Autodesk Fusion 360 part; units mm, degrees
(part 4 of 5)
  spline S17 degree 5 poles (-28.0678, -2.6304) (-28.0819, -2.6317) (-28.1102, -2.634) (-28.1526, -2.6363) (-28.2093, -2.6371) (-28.2803, -2.6353) (-28.3513, -2.6314) (-28.4224, -2.6261) (-28.4935, -2.6201) (-28.5647, -2.6137) (-28.6359, -2.6067) (-28.7071, -2.5991) (-28.7783, -2.5906) (-28.8495, -2.5811) (-28.9207, -2.5705) (-28.9919, -2.559) (-29.0631, -2.5467) (-29.1343, -2.5337) (-29.2055, -2.5201) (-29.2767, -2.5059) (-29.3478, -2.4912) (-29.419, -2.4759) (-29.4901, -2.46) (-29.5612, -2.4434) (-29.6322, -2.4261) (-29.7033, -2.4083) (-29.7743, -2.3899) (-29.8453, -2.3709) (-29.9162, -2.3515) (-29.9871, -2.3314) (-30.058, -2.3109) (-30.1288, -2.2899) (-30.1996, -2.2683) (-30.2704, -2.2463) (-30.3411, -2.2237) (-30.4117, -2.2006) (-30.4824, -2.1771) (-30.5529, -2.153) (-30.6235, -2.1285) (-30.6939, -2.1035) (-30.7644, -2.0781) (-30.8347, -2.0522) (-30.905, -2.0259) (-30.9753, -1.9991) (-31.0455, -1.9718) (-31.1156, -1.9441) (-31.1857, -1.916) (-31.2558, -1.8874) (-31.3257, -1.8584) (-31.3956, -1.829) (-31.4655, -1.7992) (-31.5352, -1.7689) (-31.6049, -1.7383) (-31.6746, -1.7072) (-31.7442, -1.6757) (-31.8137, -1.6438) (-31.8831, -1.6115) (-31.9524, -1.5788) (-32.0217, -1.5457) (-32.0909, -1.5122) (-32.1601, -1.4784) (-32.2291, -1.4441) (-32.2981, -1.4094) (-32.367, -1.3744) (-32.4359, -1.339) (-32.5046, -1.3032) (-32.5733, -1.267) (-32.6419, -1.2305) (-32.7104, -1.1936) (-32.7788, -1.1563) (-32.8471, -1.1186) (-32.9017, -1.0882) (-32.9427, -1.0652) (-32.9699, -1.0499) (-32.9835, -1.0421) knots 0 0 0 0 0 0 0.01428571 0.02857143 0.04285714 0.05714286 0.07142857 0.08571429 0.1 0.11428571 0.12857143 0.14285714 0.15714286 0.17142857 0.18571429 0.2 0.21428571 0.22857143 0.24285714 0.25714286 0.27142857 0.28571429 0.3 0.31428571 0.32857143 0.34285714 0.35714286 0.37142857 0.38571429 0.4 0.41428571 0.42857143 0.44285714 0.45714286 0.47142857 0.48571429 0.5 0.51428571 0.52857143 0.54285714 0.55714286 0.57142857 0.58571429 0.6 0.61428571 0.62857143 0.64285714 0.65714286 0.67142857 0.68571429 0.7 0.71428571 0.72857143 0.74285714 0.75714286 0.77142857 0.78571429 0.8 0.81428571 0.82857143 0.84285714 0.85714286 0.87142857 0.88571429 0.9 0.91428571 0.92857143 0.94285714 0.95714286 0.97142857 0.98571429 1 1 1 1 1 1
  line L17 (-28.0678, -2.6304) -> (-27.7691, -2.6026)
  arc A34 (-26.0521, -3.9455) -> (-27.7691, -2.6026) centre (-27.6217, -4.1832) ccw
  arc A35 (-26.0521, -3.9455) -> (-25.9963, -4.2981) centre (0, 0) ccw
  arc A36 (-27.2142, -6.1059) -> (-25.9963, -4.2981) centre (-27.5625, -4.5571) ccw
  line L18 (-27.2142, -6.1059) -> (-27.5069, -6.1717)
  spline S18 degree 5 poles (-27.5069, -6.1717) (-27.5207, -6.1748) (-27.5483, -6.1814) (-27.5894, -6.1924) (-27.6436, -6.2091) (-27.7105, -6.2328) (-27.7768, -6.2585) (-27.8428, -6.2854) (-27.9086, -6.3131) (-27.9743, -6.3412) (-28.0399, -6.3698) (-28.1052, -6.3991) (-28.1703, -6.4291) (-28.2351, -6.4602) (-28.2996, -6.4923) (-28.3637, -6.5252) (-28.4276, -6.5589) (-28.4913, -6.5933) (-28.5548, -6.6282) (-28.6182, -6.6637) (-28.6813, -6.6997) (-28.7442, -6.7362) (-28.8069, -6.7734) (-28.8694, -6.8111) (-28.9317, -6.8495) (-28.9937, -6.8884) (-29.0556, -6.9278) (-29.1172, -6.9678) (-29.1786, -7.0083) (-29.2399, -7.0492) (-29.301, -7.0906) (-29.3618, -7.1325) (-29.4225, -7.1749) (-29.483, -7.2177) (-29.5432, -7.261) (-29.6033, -7.3048) (-29.6632, -7.3491) (-29.7229, -7.3937) (-29.7824, -7.4388) (-29.8417, -7.4844) (-29.9008, -7.5303) (-29.9597, -7.5767) (-30.0185, -7.6235) (-30.077, -7.6707) (-30.1353, -7.7183) (-30.1935, -7.7663) (-30.2515, -7.8147) (-30.3092, -7.8635) (-30.3668, -7.9127) (-30.4242, -7.9623) (-30.4814, -8.0122) (-30.5384, -8.0626) (-30.5952, -8.1133) (-30.6519, -8.1644) (-30.7083, -8.2158) (-30.7645, -8.2676) (-30.8206, -8.3198) (-30.8765, -8.3723) (-30.9321, -8.4252) (-30.9876, -8.4784) (-31.0429, -8.532) (-31.098, -8.5859) (-31.1529, -8.6402) (-31.2076, -8.6948) (-31.2621, -8.7498) (-31.3164, -8.8051) (-31.3706, -8.8607) (-31.4245, -8.9166) (-31.4783, -8.9729) (-31.5318, -9.0295) (-31.5852, -9.0864) (-31.6277, -9.1322) (-31.6595, -9.1667) (-31.6807, -9.1898) (-31.6913, -9.2013) knots 0 0 0 0 0 0 0.01428571 0.02857143 0.04285714 0.05714286 0.07142857 0.08571429 0.1 0.11428571 0.12857143 0.14285714 0.15714286 0.17142857 0.18571429 0.2 0.21428571 0.22857143 0.24285714 0.25714286 0.27142857 0.28571429 0.3 0.31428571 0.32857143 0.34285714 0.35714286 0.37142857 0.38571429 0.4 0.41428571 0.42857143 0.44285714 0.45714286 0.47142857 0.48571429 0.5 0.51428571 0.52857143 0.54285714 0.55714286 0.57142857 0.58571429 0.6 0.61428571 0.62857143 0.64285714 0.65714286 0.67142857 0.68571429 0.7 0.71428571 0.72857143 0.74285714 0.75714286 0.77142857 0.78571429 0.8 0.81428571 0.82857143 0.84285714 0.85714286 0.87142857 0.88571429 0.9 0.91428571 0.92857143 0.94285714 0.95714286 0.97142857 0.98571429 1 1 1 1 1 1
  arc A37 (-31.6913, -9.2013) -> (-31.0472, -11.1836) centre (0, 0) ccw
  spline S19 degree 5 poles (-25.8812, -11.1751) (-25.8942, -11.1807) (-25.9204, -11.1916) (-25.9601, -11.2069) (-26.0137, -11.2252) (-26.0818, -11.2454) (-26.1506, -11.2636) (-26.2198, -11.2806) (-26.2893, -11.2969) (-26.359, -11.3128) (-26.4288, -11.3281) (-26.4989, -11.3429) (-26.5692, -11.3568) (-26.6399, -11.3697) (-26.7109, -11.3817) (-26.7822, -11.3928) (-26.8537, -11.4031) (-26.9254, -11.4127) (-26.9973, -11.4218) (-27.0694, -11.4303) (-27.1416, -11.4383) (-27.214, -11.4457) (-27.2866, -11.4525) (-27.3593, -11.4587) (-27.4322, -11.4643) (-27.5053, -11.4693) (-27.5785, -11.4737) (-27.6519, -11.4776) (-27.7254, -11.481) (-27.799, -11.4839) (-27.8727, -11.4863) (-27.9466, -11.4881) (-28.0206, -11.4895) (-28.0947, -11.4904) (-28.1689, -11.4908) (-28.2433, -11.4907) (-28.3177, -11.4901) (-28.3922, -11.489) (-28.4669, -11.4875) (-28.5416, -11.4855) (-28.6165, -11.4831) (-28.6914, -11.4802) (-28.7664, -11.4769) (-28.8415, -11.4731) (-28.9167, -11.4689) (-28.992, -11.4642) (-29.0673, -11.4591) (-29.1427, -11.4536) (-29.2182, -11.4477) (-29.2938, -11.4413) (-29.3695, -11.4345) (-29.4452, -11.4273) (-29.5209, -11.4196) (-29.5968, -11.4116) (-29.6727, -11.4032) (-29.7486, -11.3943) (-29.8246, -11.385) (-29.9007, -11.3754) (-29.9768, -11.3653) (-30.053, -11.3549) (-30.1292, -11.344) (-30.2055, -11.3328) (-30.2818, -11.3211) (-30.3582, -11.3091) (-30.4346, -11.2967) (-30.511, -11.2839) (-30.5875, -11.2707) (-30.664, -11.2572) (-30.7406, -11.2432) (-30.8172, -11.2289) (-30.8938, -11.2142) (-30.9551, -11.2022) (-31.0011, -11.193) (-31.0318, -11.1867) (-31.0472, -11.1836) knots 0 0 0 0 0 0 0.01428571 0.02857143 0.04285714 0.05714286 0.07142857 0.08571429 0.1 0.11428571 0.12857143 0.14285714 0.15714286 0.17142857 0.18571429 0.2 0.21428571 0.22857143 0.24285714 0.25714286 0.27142857 0.28571429 0.3 0.31428571 0.32857143 0.34285714 0.35714286 0.37142857 0.38571429 0.4 0.41428571 0.42857143 0.44285714 0.45714286 0.47142857 0.48571429 0.5 0.51428571 0.52857143 0.54285714 0.55714286 0.57142857 0.58571429 0.6 0.61428571 0.62857143 0.64285714 0.65714286 0.67142857 0.68571429 0.7 0.71428571 0.72857143 0.74285714 0.75714286 0.77142857 0.78571429 0.8 0.81428571 0.82857143 0.84285714 0.85714286 0.87142857 0.88571429 0.9 0.91428571 0.92857143 0.94285714 0.95714286 0.97142857 0.98571429 1 1 1 1 1 1
  line L19 (-25.8812, -11.1751) -> (-25.6057, -11.0563)
  arc A38 (-23.5578, -11.803) -> (-25.6057, -11.0563) centre (-24.9771, -12.5141) ccw
  arc A39 (-23.5578, -11.803) -> (-23.3957, -12.1211) centre (0, 0) ccw
  arc A40 (-23.9954, -14.2167) -> (-23.3957, -12.1211) centre (-24.8053, -12.8513) ccw
  line L20 (-23.9954, -14.2167) -> (-24.2534, -14.3698)
  spline S20 degree 5 poles (-24.2534, -14.3698) (-24.2657, -14.377) (-24.2899, -14.3918) (-24.3255, -14.4149) (-24.3719, -14.4475) (-24.4282, -14.4907) (-24.4834, -14.5357) (-24.5378, -14.5817) (-24.5918, -14.6283) (-24.6456, -14.6754) (-24.6991, -14.7228) (-24.7522, -14.7709) (-24.8048, -14.8196) (-24.8568, -14.8691) (-24.9083, -14.9195) (-24.9591, -14.9707) (-25.0095, -15.0225) (-25.0594, -15.0749) (-25.109, -15.1278) (-25.1583, -15.1811) (-25.2072, -15.2348) (-25.2557, -15.289) (-25.3039, -15.3437) (-25.3517, -15.3989) (-25.399, -15.4546) (-25.446, -15.5108) (-25.4927, -15.5674) (-25.5389, -15.6245) (-25.5849, -15.6819) (-25.6305, -15.7398) (-25.6758, -15.7981) (-25.7207, -15.8567) (-25.7653, -15.9158) (-25.8096, -15.9752) (-25.8535, -16.035) (-25.8971, -16.0952) (-25.9404, -16.1558) (-25.9834, -16.2167) (-26.026, -16.278) (-26.0683, -16.3396) (-26.1104, -16.4016) (-26.1521, -16.4639) (-26.1935, -16.5266) (-26.2346, -16.5896) (-26.2753, -16.6529) (-26.3158, -16.7165) (-26.356, -16.7804) (-26.3958, -16.8447) (-26.4354, -16.9093) (-26.4747, -16.9742) (-26.5136, -17.0394) (-26.5523, -17.1048) (-26.5907, -17.1706) (-26.6287, -17.2367) (-26.6665, -17.3031) (-26.704, -17.3697) (-26.7412, -17.4367) (-26.7781, -17.5039) (-26.8147, -17.5714) (-26.851, -17.6392) (-26.887, -17.7072) (-26.9227, -17.7755) (-26.9582, -17.8441) (-26.9933, -17.913) (-27.0282, -17.9821) (-27.0628, -18.0514) (-27.0971, -18.1211) (-27.1311, -18.1909) (-27.1648, -18.2611) (-27.1983, -18.3314) (-27.2314, -18.4021) (-27.2577, -18.4588) (-27.2773, -18.5014) (-27.2903, -18.5299) (-27.2968, -18.5441) knots 0 0 0 0 0 0 0.01428571 0.02857143 0.04285714 0.05714286 0.07142857 0.08571429 0.1 0.11428571 0.12857143 0.14285714 0.15714286 0.17142857 0.18571429 0.2 0.21428571 0.22857143 0.24285714 0.25714286 0.27142857 0.28571429 0.3 0.31428571 0.32857143 0.34285714 0.35714286 0.37142857 0.38571429 0.4 0.41428571 0.42857143 0.44285714 0.45714286 0.47142857 0.48571429 0.5 0.51428571 0.52857143 0.54285714 0.55714286 0.57142857 0.58571429 0.6 0.61428571 0.62857143 0.64285714 0.65714286 0.67142857 0.68571429 0.7 0.71428571 0.72857143 0.74285714 0.75714286 0.77142857 0.78571429 0.8 0.81428571 0.82857143 0.84285714 0.85714286 0.87142857 0.88571429 0.9 0.91428571 0.92857143 0.94285714 0.95714286 0.97142857 0.98571429 1 1 1 1 1 1
  arc A41 (-27.2968, -18.5441) -> (-26.0717, -20.2304) centre (0, 0) ccw
  spline S21 degree 5 poles (-21.1612, -18.6259) (-21.1718, -18.6353) (-21.1934, -18.6537) (-21.2264, -18.6805) (-21.2717, -18.7145) (-21.3302, -18.7547) (-21.39, -18.7933) (-21.4506, -18.8308) (-21.5117, -18.8678) (-21.573, -18.9044) (-21.6347, -18.9407) (-21.6968, -18.9763) (-21.7594, -19.0113) (-21.8226, -19.0454) (-21.8864, -19.0788) (-21.9508, -19.1113) (-22.0156, -19.1432) (-22.0809, -19.1745) (-22.1465, -19.2054) (-22.2124, -19.2358) (-22.2786, -19.2657) (-22.3452, -19.2951) (-22.4121, -19.324) (-22.4793, -19.3523) (-22.5469, -19.3802) (-22.6149, -19.4075) (-22.6832, -19.4344) (-22.7517, -19.4607) (-22.8206, -19.4867) (-22.8897, -19.5122) (-22.9591, -19.5372) (-23.0288, -19.5618) (-23.0987, -19.586) (-23.1689, -19.6098) (-23.2394, -19.6331) (-23.3101, -19.6559) (-23.3811, -19.6784) (-23.4523, -19.7004) (-23.5238, -19.722) (-23.5955, -19.7432) (-23.6674, -19.7641) (-23.7396, -19.7845) (-23.8119, -19.8045) (-23.8845, -19.8241) (-23.9573, -19.8433) (-24.0304, -19.8621) (-24.1036, -19.8806) (-24.177, -19.8986) (-24.2507, -19.9163) (-24.3245, -19.9336) (-24.3986, -19.9505) (-24.4728, -19.967) (-24.5472, -19.9832) (-24.6218, -19.999) (-24.6966, -20.0144) (-24.7716, -20.0295) (-24.8467, -20.0441) (-24.9221, -20.0585) (-24.9976, -20.0724) (-25.0733, -20.086) (-25.1491, -20.0992) (-25.2251, -20.1121) (-25.3013, -20.1246) (-25.3776, -20.1368) (-25.4541, -20.1486) (-25.5308, -20.16) (-25.6076, -20.1711) (-25.6846, -20.1819) (-25.7617, -20.1923) (-25.839, -20.2024) (-25.9164, -20.2121) (-25.9784, -20.2196) (-26.025, -20.225) (-26.0561, -20.2286) (-26.0717, -20.2304) knots 0 0 0 0 0 0 0.01428571 0.02857143 0.04285714 0.05714286 0.07142857 0.08571429 0.1 0.11428571 0.12857143 0.14285714 0.15714286 0.17142857 0.18571429 0.2 0.21428571 0.22857143 0.24285714 0.25714286 0.27142857 0.28571429 0.3 0.31428571 0.32857143 0.34285714 0.35714286 0.37142857 0.38571429 0.4 0.41428571 0.42857143 0.44285714 0.45714286 0.47142857 0.48571429 0.5 0.51428571 0.52857143 0.54285714 0.55714286 0.57142857 0.58571429 0.6 0.61428571 0.62857143 0.64285714 0.65714286 0.67142857 0.68571429 0.7 0.71428571 0.72857143 0.74285714 0.75714286 0.77142857 0.78571429 0.8 0.81428571 0.82857143 0.84285714 0.85714286 0.87142857 0.88571429 0.9 0.91428571 0.92857143 0.94285714 0.95714286 0.97142857 0.98571429 1 1 1 1 1 1
  line L21 (-21.1612, -18.6259) -> (-20.9359, -18.4278)
  arc A42 (-18.7575, -18.5051) -> (-20.9359, -18.4278) centre (-19.8876, -19.62) ccw
  arc A43 (-18.7575, -18.5051) -> (-18.5051, -18.7575) centre (0, 0) ccw
  arc A44 (-18.4278, -20.9359) -> (-18.5051, -18.7575) centre (-19.62, -19.8876) ccw
  line L22 (-18.4278, -20.9359) -> (-18.6259, -21.1612)
  spline S22 degree 5 poles (-18.6259, -21.1612) (-18.6353, -21.1718) (-18.6537, -21.1934) (-18.6805, -21.2264) (-18.7145, -21.2717) (-18.7547, -21.3302) (-18.7933, -21.39) (-18.8308, -21.4506) (-18.8678, -21.5117) (-18.9044, -21.573) (-18.9407, -21.6347) (-18.9763, -21.6968) (-19.0113, -21.7594) (-19.0454, -21.8226) (-19.0788, -21.8864) (-19.1113, -21.9508) (-19.1432, -22.0156) (-19.1745, -22.0809) (-19.2054, -22.1465) (-19.2358, -22.2124) (-19.2657, -22.2786) (-19.2951, -22.3452) (-19.324, -22.4121) (-19.3523, -22.4793) (-19.3802, -22.5469) (-19.4075, -22.6149) (-19.4344, -22.6832) (-19.4607, -22.7517) (-19.4867, -22.8206) (-19.5122, -22.8897) (-19.5372, -22.9591) (-19.5618, -23.0288) (-19.586, -23.0987) (-19.6098, -23.1689) (-19.6331, -23.2394) (-19.6559, -23.3101) (-19.6784, -23.3811) (-19.7004, -23.4523) (-19.722, -23.5238) (-19.7432, -23.5955) (-19.7641, -23.6674) (-19.7845, -23.7396) (-19.8045, -23.8119) (-19.8241, -23.8845) (-19.8433, -23.9573) (-19.8621, -24.0304) (-19.8806, -24.1036) (-19.8986, -24.177) (-19.9163, -24.2507) (-19.9336, -24.3245) (-19.9505, -24.3986) (-19.967, -24.4728) (-19.9832, -24.5472) (-19.999, -24.6218) (-20.0144, -24.6966) (-20.0295, -24.7716) (-20.0441, -24.8467) (-20.0585, -24.9221) (-20.0724, -24.9976) (-20.086, -25.0733) (-20.0992, -25.1491) (-20.1121, -25.2251) (-20.1246, -25.3013) (-20.1368, -25.3776) (-20.1486, -25.4541) (-20.16, -25.5308) (-20.1711, -25.6076) (-20.1819, -25.6846) (-20.1923, -25.7617) (-20.2024, -25.839) (-20.2121, -25.9164) (-20.2196, -25.9784) (-20.225, -26.025) (-20.2286, -26.0561) (-20.2304, -26.0717) knots 0 0 0 0 0 0 0.01428571 0.02857143 0.04285714 0.05714286 0.07142857 0.08571429 0.1 0.11428571 0.12857143 0.14285714 0.15714286 0.17142857 0.18571429 0.2 0.21428571 0.22857143 0.24285714 0.25714286 0.27142857 0.28571429 0.3 0.31428571 0.32857143 0.34285714 0.35714286 0.37142857 0.38571429 0.4 0.41428571 0.42857143 0.44285714 0.45714286 0.47142857 0.48571429 0.5 0.51428571 0.52857143 0.54285714 0.55714286 0.57142857 0.58571429 0.6 0.61428571 0.62857143 0.64285714 0.65714286 0.67142857 0.68571429 0.7 0.71428571 0.72857143 0.74285714 0.75714286 0.77142857 0.78571429 0.8 0.81428571 0.82857143 0.84285714 0.85714286 0.87142857 0.88571429 0.9 0.91428571 0.92857143 0.94285714 0.95714286 0.97142857 0.98571429 1 1 1 1 1 1
  arc A45 (-20.2304, -26.0717) -> (-18.5441, -27.2968) centre (0, 0) ccw
  spline S23 degree 5 poles (-14.3698, -24.2534) (-14.377, -24.2657) (-14.3918, -24.2899) (-14.4149, -24.3255) (-14.4475, -24.3719) (-14.4907, -24.4282) (-14.5357, -24.4834) (-14.5817, -24.5378) (-14.6283, -24.5918) (-14.6754, -24.6456) (-14.7228, -24.6991) (-14.7709, -24.7522) (-14.8196, -24.8048) (-14.8691, -24.8568) (-14.9195, -24.9083) (-14.9707, -24.9591) (-15.0225, -25.0095) (-15.0749, -25.0594) (-15.1278, -25.109) (-15.1811, -25.1583) (-15.2348, -25.2072) (-15.289, -25.2557) (-15.3437, -25.3039) (-15.3989, -25.3517) (-15.4546, -25.399) (-15.5108, -25.446) (-15.5674, -25.4927) (-15.6245, -25.5389) (-15.6819, -25.5849) (-15.7398, -25.6305) (-15.7981, -25.6758) (-15.8567, -25.7207) (-15.9158, -25.7653) (-15.9752, -25.8096) (-16.035, -25.8535) (-16.0952, -25.8971) (-16.1558, -25.9404) (-16.2167, -25.9834) (-16.278, -26.026) (-16.3396, -26.0683) (-16.4016, -26.1104) (-16.4639, -26.1521) (-16.5266, -26.1935) (-16.5896, -26.2346) (-16.6529, -26.2753) (-16.7165, -26.3158) (-16.7804, -26.356) (-16.8447, -26.3958) (-16.9093, -26.4354) (-16.9742, -26.4747) (-17.0394, -26.5136) (-17.1048, -26.5523) (-17.1706, -26.5907) (-17.2367, -26.6287) (-17.3031, -26.6665) (-17.3697, -26.704) (-17.4367, -26.7412) (-17.5039, -26.7781) (-17.5714, -26.8147) (-17.6392, -26.851) (-17.7072, -26.887) (-17.7755, -26.9227) (-17.8441, -26.9582) (-17.913, -26.9933) (-17.9821, -27.0282) (-18.0514, -27.0628) (-18.1211, -27.0971) (-18.1909, -27.1311) (-18.2611, -27.1648) (-18.3314, -27.1983) (-18.4021, -27.2314) (-18.4588, -27.2577) (-18.5014, -27.2773) (-18.5299, -27.2903) (-18.5441, -27.2968) knots 0 0 0 0 0 0 0.01428571 0.02857143 0.04285714 0.05714286 0.07142857 0.08571429 0.1 0.11428571 0.12857143 0.14285714 0.15714286 0.17142857 0.18571429 0.2 0.21428571 0.22857143 0.24285714 0.25714286 0.27142857 0.28571429 0.3 0.31428571 0.32857143 0.34285714 0.35714286 0.37142857 0.38571429 0.4 0.41428571 0.42857143 0.44285714 0.45714286 0.47142857 0.48571429 0.5 0.51428571 0.52857143 0.54285714 0.55714286 0.57142857 0.58571429 0.6 0.61428571 0.62857143 0.64285714 0.65714286 0.67142857 0.68571429 0.7 0.71428571 0.72857143 0.74285714 0.75714286 0.77142857 0.78571429 0.8 0.81428571 0.82857143 0.84285714 0.85714286 0.87142857 0.88571429 0.9 0.91428571 0.92857143 0.94285714 0.95714286 0.97142857 0.98571429 1 1 1 1 1 1
  line L23 (-14.3698, -24.2534) -> (-14.2167, -23.9954)
  arc A46 (-12.1211, -23.3957) -> (-14.2167, -23.9954) centre (-12.8513, -24.8053) ccw
  arc A47 (-12.1211, -23.3957) -> (-11.803, -23.5578) centre (0, 0) ccw
  arc A48 (-11.0563, -25.6057) -> (-11.803, -23.5578) centre (-12.5141, -24.9771) ccw
  line L24 (-11.0563, -25.6057) -> (-11.1751, -25.8812)
  spline S24 degree 5 poles (-11.1751, -25.8812) (-11.1807, -25.8942) (-11.1916, -25.9204) (-11.2069, -25.9601) (-11.2252, -26.0137) (-11.2454, -26.0818) (-11.2636, -26.1506) (-11.2806, -26.2198) (-11.2969, -26.2893) (-11.3128, -26.359) (-11.3281, -26.4288) (-11.3429, -26.4989) (-11.3568, -26.5692) (-11.3697, -26.6399) (-11.3817, -26.7109) (-11.3928, -26.7822) (-11.4031, -26.8537) (-11.4127, -26.9254) (-11.4218, -26.9973) (-11.4303, -27.0694) (-11.4383, -27.1416) (-11.4457, -27.214) (-11.4525, -27.2866) (-11.4587, -27.3593) (-11.4643, -27.4322) (-11.4693, -27.5053) (-11.4737, -27.5785) (-11.4776, -27.6519) (-11.481, -27.7254) (-11.4839, -27.799) (-11.4863, -27.8727) (-11.4881, -27.9466) (-11.4895, -28.0206) (-11.4904, -28.0947) (-11.4908, -28.1689) (-11.4907, -28.2433) (-11.4901, -28.3177) (-11.489, -28.3922) (-11.4875, -28.4669) (-11.4855, -28.5416) (-11.4831, -28.6165) (-11.4802, -28.6914) (-11.4769, -28.7664) (-11.4731, -28.8415) (-11.4689, -28.9167) (-11.4642, -28.992) (-11.4591, -29.0673) (-11.4536, -29.1427) (-11.4477, -29.2182) (-11.4413, -29.2938) (-11.4345, -29.3695) (-11.4273, -29.4452) (-11.4196, -29.5209) (-11.4116, -29.5968) (-11.4032, -29.6727) (-11.3943, -29.7486) (-11.385, -29.8246) (-11.3754, -29.9007) (-11.3653, -29.9768) (-11.3549, -30.053) (-11.344, -30.1292) (-11.3328, -30.2055) (-11.3211, -30.2818) (-11.3091, -30.3582) (-11.2967, -30.4346) (-11.2839, -30.511) (-11.2707, -30.5875) (-11.2572, -30.664) (-11.2432, -30.7406) (-11.2289, -30.8172) (-11.2142, -30.8938) (-11.2022, -30.9551) (-11.193, -31.0011) (-11.1867, -31.0318) (-11.1836, -31.0472) knots 0 0 0 0 0 0 0.01428571 0.02857143 0.04285714 0.05714286 0.07142857 0.08571429 0.1 0.11428571 0.12857143 0.14285714 0.15714286 0.17142857 0.18571429 0.2 0.21428571 0.22857143 0.24285714 0.25714286 0.27142857 0.28571429 0.3 0.31428571 0.32857143 0.34285714 0.35714286 0.37142857 0.38571429 0.4 0.41428571 0.42857143 0.44285714 0.45714286 0.47142857 0.48571429 0.5 0.51428571 0.52857143 0.54285714 0.55714286 0.57142857 0.58571429 0.6 0.61428571 0.62857143 0.64285714 0.65714286 0.67142857 0.68571429 0.7 0.71428571 0.72857143 0.74285714 0.75714286 0.77142857 0.78571429 0.8 0.81428571 0.82857143 0.84285714 0.85714286 0.87142857 0.88571429 0.9 0.91428571 0.92857143 0.94285714 0.95714286 0.97142857 0.98571429 1 1 1 1 1 1
  arc A49 (-11.1836, -31.0472) -> (-9.2013, -31.6913) centre (0, 0) ccw
  spline S25 degree 5 poles (-6.1717, -27.5069) (-6.1748, -27.5207) (-6.1814, -27.5483) (-6.1924, -27.5894) (-6.2091, -27.6436) (-6.2328, -27.7105) (-6.2585, -27.7768) (-6.2854, -27.8428) (-6.3131, -27.9086) (-6.3412, -27.9743) (-6.3698, -28.0399) (-6.3991, -28.1052) (-6.4291, -28.1703) (-6.4602, -28.2351) (-6.4923, -28.2996) (-6.5252, -28.3637) (-6.5589, -28.4276) (-6.5933, -28.4913) (-6.6282, -28.5548) (-6.6637, -28.6182) (-6.6997, -28.6813) (-6.7362, -28.7442) (-6.7734, -28.8069) (-6.8111, -28.8694) (-6.8495, -28.9317) (-6.8884, -28.9937) (-6.9278, -29.0556) (-6.9678, -29.1172) (-7.0083, -29.1786) (-7.0492, -29.2399) (-7.0906, -29.301) (-7.1325, -29.3618) (-7.1749, -29.4225) (-7.2177, -29.483) (-7.261, -29.5432) (-7.3048, -29.6033) (-7.3491, -29.6632) (-7.3937, -29.7229) (-7.4388, -29.7824) (-7.4844, -29.8417) (-7.5303, -29.9008) (-7.5767, -29.9597) (-7.6235, -30.0185) (-7.6707, -30.077) (-7.7183, -30.1353) (-7.7663, -30.1935) (-7.8147, -30.2515) (-7.8635, -30.3092) (-7.9127, -30.3668) (-7.9623, -30.4242) (-8.0122, -30.4814) (-8.0626, -30.5384) (-8.1133, -30.5952) (-8.1644, -30.6519) (-8.2158, -30.7083) (-8.2676, -30.7645) (-8.3198, -30.8206) (-8.3723, -30.8765) (-8.4252, -30.9321) (-8.4784, -30.9876) (-8.532, -31.0429) (-8.5859, -31.098) (-8.6402, -31.1529) (-8.6948, -31.2076) (-8.7498, -31.2621) (-8.8051, -31.3164) (-8.8607, -31.3706) (-8.9166, -31.4245) (-8.9729, -31.4783) (-9.0295, -31.5318) (-9.0864, -31.5852) (-9.1322, -31.6277) (-9.1667, -31.6595) (-9.1898, -31.6807) (-9.2013, -31.6913) knots 0 0 0 0 0 0 0.01428571 0.02857143 0.04285714 0.05714286 0.07142857 0.08571429 0.1 0.11428571 0.12857143 0.14285714 0.15714286 0.17142857 0.18571429 0.2 0.21428571 0.22857143 0.24285714 0.25714286 0.27142857 0.28571429 0.3 0.31428571 0.32857143 0.34285714 0.35714286 0.37142857 0.38571429 0.4 0.41428571 0.42857143 0.44285714 0.45714286 0.47142857 0.48571429 0.5 0.51428571 0.52857143 0.54285714 0.55714286 0.57142857 0.58571429 0.6 0.61428571 0.62857143 0.64285714 0.65714286 0.67142857 0.68571429 0.7 0.71428571 0.72857143 0.74285714 0.75714286 0.77142857 0.78571429 0.8 0.81428571 0.82857143 0.84285714 0.85714286 0.87142857 0.88571429 0.9 0.91428571 0.92857143 0.94285714 0.95714286 0.97142857 0.98571429 1 1 1 1 1 1
  line L25 (-6.1717, -27.5069) -> (-6.1059, -27.2142)
  arc A50 (-4.2981, -25.9963) -> (-6.1059, -27.2142) centre (-4.5571, -27.5625) ccw
  arc A51 (-4.2981, -25.9963) -> (-3.9455, -26.0521) centre (0, 0) ccw
  arc A52 (-2.6026, -27.7691) -> (-3.9455, -26.0521) centre (-4.1832, -27.6217) ccw
  line L26 (-2.6026, -27.7691) -> (-2.6304, -28.0678)
  spline S26 degree 5 poles (-2.6304, -28.0678) (-2.6317, -28.0819) (-2.634, -28.1102) (-2.6363, -28.1526) (-2.6371, -28.2093) (-2.6353, -28.2803) (-2.6314, -28.3513) (-2.6261, -28.4224) (-2.6201, -28.4935) (-2.6137, -28.5647) (-2.6067, -28.6359) (-2.5991, -28.7071) (-2.5906, -28.7783) (-2.5811, -28.8495) (-2.5705, -28.9207) (-2.559, -28.9919) (-2.5467, -29.0631) (-2.5337, -29.1343) (-2.5201, -29.2055) (-2.5059, -29.2767) (-2.4912, -29.3478) (-2.4759, -29.419) (-2.46, -29.4901) (-2.4434, -29.5612) (-2.4261, -29.6322) (-2.4083, -29.7033) (-2.3899, -29.7743) (-2.3709, -29.8453) (-2.3515, -29.9162) (-2.3314, -29.9871) (-2.3109, -30.058) (-2.2899, -30.1288) (-2.2683, -30.1996) (-2.2463, -30.2704) (-2.2237, -30.3411) (-2.2006, -30.4117) (-2.1771, -30.4824) (-2.153, -30.5529) (-2.1285, -30.6235) (-2.1035, -30.6939) (-2.0781, -30.7644) (-2.0522, -30.8347) (-2.0259, -30.905) (-1.9991, -30.9753) (-1.9718, -31.0455) (-1.9441, -31.1156) (-1.916, -31.1857) (-1.8874, -31.2558) (-1.8584, -31.3257) (-1.829, -31.3956) (-1.7992, -31.4655) (-1.7689, -31.5352) (-1.7383, -31.6049) (-1.7072, -31.6746) (-1.6757, -31.7442) (-1.6438, -31.8137) (-1.6115, -31.8831) (-1.5788, -31.9524) (-1.5457, -32.0217) (-1.5122, -32.0909) (-1.4784, -32.1601) (-1.4441, -32.2291) (-1.4094, -32.2981) (-1.3744, -32.367) (-1.339, -32.4359) (-1.3032, -32.5046) (-1.267, -32.5733) (-1.2305, -32.6419) (-1.1936, -32.7104) (-1.1563, -32.7788) (-1.1186, -32.8471) (-1.0882, -32.9017) (-1.0652, -32.9427) (-1.0499, -32.9699) (-1.0421, -32.9835) knots 0 0 0 0 0 0 0.01428571 0.02857143 0.04285714 0.05714286 0.07142857 0.08571429 0.1 0.11428571 0.12857143 0.14285714 0.15714286 0.17142857 0.18571429 0.2 0.21428571 0.22857143 0.24285714 0.25714286 0.27142857 0.28571429 0.3 0.31428571 0.32857143 0.34285714 0.35714286 0.37142857 0.38571429 0.4 0.41428571 0.42857143 0.44285714 0.45714286 0.47142857 0.48571429 0.5 0.51428571 0.52857143 0.54285714 0.55714286 0.57142857 0.58571429 0.6 0.61428571 0.62857143 0.64285714 0.65714286 0.67142857 0.68571429 0.7 0.71428571 0.72857143 0.74285714 0.75714286 0.77142857 0.78571429 0.8 0.81428571 0.82857143 0.84285714 0.85714286 0.87142857 0.88571429 0.9 0.91428571 0.92857143 0.94285714 0.95714286 0.97142857 0.98571429 1 1 1 1 1 1
  arc A53 (-1.0421, -32.9835) -> (1.0421, -32.9835) centre (0, 0) ccw
  spline S27 degree 5 poles (2.6304, -28.0678) (2.6317, -28.0819) (2.634, -28.1102) (2.6363, -28.1526) (2.6371, -28.2093) (2.6353, -28.2803) (2.6314, -28.3513) (2.6261, -28.4224) (2.6201, -28.4935) (2.6137, -28.5647) (2.6067, -28.6359) (2.5991, -28.7071) (2.5906, -28.7783) (2.5811, -28.8495) (2.5705, -28.9207) (2.559, -28.9919) (2.5467, -29.0631) (2.5337, -29.1343) (2.5201, -29.2055) (2.5059, -29.2767) (2.4912, -29.3478) (2.4759, -29.419) (2.46, -29.4901) (2.4434, -29.5612) (2.4261, -29.6322) (2.4083, -29.7033) (2.3899, -29.7743) (2.3709, -29.8453) (2.3515, -29.9162) (2.3314, -29.9871) (2.3109, -30.058) (2.2899, -30.1288) (2.2683, -30.1996) (2.2463, -30.2704) (2.2237, -30.3411) (2.2006, -30.4117) (2.1771, -30.4824) (2.153, -30.5529) (2.1285, -30.6235) (2.1035, -30.6939) (2.0781, -30.7644) (2.0522, -30.8347) (2.0259, -30.905) (1.9991, -30.9753) (1.9718, -31.0455) (1.9441, -31.1156) (1.916, -31.1857) (1.8874, -31.2558) (1.8584, -31.3257) (1.829, -31.3956) (1.7992, -31.4655) (1.7689, -31.5352) (1.7383, -31.6049) (1.7072, -31.6746) (1.6757, -31.7442) (1.6438, -31.8137) (1.6115, -31.8831) (1.5788, -31.9524) (1.5457, -32.0217) (1.5122, -32.0909) (1.4784, -32.1601) (1.4441, -32.2291) (1.4094, -32.2981) (1.3744, -32.367) (1.339, -32.4359) (1.3032, -32.5046) (1.267, -32.5733) (1.2305, -32.6419) (1.1936, -32.7104) (1.1563, -32.7788) (1.1186, -32.8471) (1.0882, -32.9017) (1.0652, -32.9427) (1.0499, -32.9699) (1.0421, -32.9835) knots 0 0 0 0 0 0 0.01428571 0.02857143 0.04285714 0.05714286 0.07142857 0.08571429 0.1 0.11428571 0.12857143 0.14285714 0.15714286 0.17142857 0.18571429 0.2 0.21428571 0.22857143 0.24285714 0.25714286 0.27142857 0.28571429 0.3 0.31428571 0.32857143 0.34285714 0.35714286 0.37142857 0.38571429 0.4 0.41428571 0.42857143 0.44285714 0.45714286 0.47142857 0.48571429 0.5 0.51428571 0.52857143 0.54285714 0.55714286 0.57142857 0.58571429 0.6 0.61428571 0.62857143 0.64285714 0.65714286 0.67142857 0.68571429 0.7 0.71428571 0.72857143 0.74285714 0.75714286 0.77142857 0.78571429 0.8 0.81428571 0.82857143 0.84285714 0.85714286 0.87142857 0.88571429 0.9 0.91428571 0.92857143 0.94285714 0.95714286 0.97142857 0.98571429 1 1 1 1 1 1
  line L27 (2.6304, -28.0678) -> (2.6026, -27.7691)
  arc A54 (3.9455, -26.0521) -> (2.6026, -27.7691) centre (4.1832, -27.6217) ccw
  arc A55 (3.9455, -26.0521) -> (4.2981, -25.9963) centre (0, 0) ccw
  arc A56 (6.1059, -27.2142) -> (4.2981, -25.9963) centre (4.5571, -27.5625) ccw
  line L28 (6.1059, -27.2142) -> (6.1717, -27.5069)
  spline S28 degree 5 poles (6.1717, -27.5069) (6.1748, -27.5207) (6.1814, -27.5483) (6.1924, -27.5894) (6.2091, -27.6436) (6.2328, -27.7105) (6.2585, -27.7768) (6.2854, -27.8428) (6.3131, -27.9086) (6.3412, -27.9743) (6.3698, -28.0399) (6.3991, -28.1052) (6.4291, -28.1703) (6.4602, -28.2351) (6.4923, -28.2996) (6.5252, -28.3637) (6.5589, -28.4276) (6.5933, -28.4913) (6.6282, -28.5548) (6.6637, -28.6182) (6.6997, -28.6813) (6.7362, -28.7442) (6.7734, -28.8069) (6.8111, -28.8694) (6.8495, -28.9317) (6.8884, -28.9937) (6.9278, -29.0556) (6.9678, -29.1172) (7.0083, -29.1786) (7.0492, -29.2399) (7.0906, -29.301) (7.1325, -29.3618) (7.1749, -29.4225) (7.2177, -29.483) (7.261, -29.5432) (7.3048, -29.6033) (7.3491, -29.6632) (7.3937, -29.7229) (7.4388, -29.7824) (7.4844, -29.8417) (7.5303, -29.9008) (7.5767, -29.9597) (7.6235, -30.0185) (7.6707, -30.077) (7.7183, -30.1353) (7.7663, -30.1935) (7.8147, -30.2515) (7.8635, -30.3092) (7.9127, -30.3668) (7.9623, -30.4242) (8.0122, -30.4814) (8.0626, -30.5384) (8.1133, -30.5952) (8.1644, -30.6519) (8.2158, -30.7083) (8.2676, -30.7645) (8.3198, -30.8206) (8.3723, -30.8765) (8.4252, -30.9321) (8.4784, -30.9876) (8.532, -31.0429) (8.5859, -31.098) (8.6402, -31.1529) (8.6948, -31.2076) (8.7498, -31.2621) (8.8051, -31.3164) (8.8607, -31.3706) (8.9166, -31.4245) (8.9729, -31.4783) (9.0295, -31.5318) (9.0864, -31.5852) (9.1322, -31.6277) (9.1667, -31.6595) (9.1898, -31.6807) (9.2013, -31.6913) knots 0 0 0 0 0 0 0.01428571 0.02857143 0.04285714 0.05714286 0.07142857 0.08571429 0.1 0.11428571 0.12857143 0.14285714 0.15714286 0.17142857 0.18571429 0.2 0.21428571 0.22857143 0.24285714 0.25714286 0.27142857 0.28571429 0.3 0.31428571 0.32857143 0.34285714 0.35714286 0.37142857 0.38571429 0.4 0.41428571 0.42857143 0.44285714 0.45714286 0.47142857 0.48571429 0.5 0.51428571 0.52857143 0.54285714 0.55714286 0.57142857 0.58571429 0.6 0.61428571 0.62857143 0.64285714 0.65714286 0.67142857 0.68571429 0.7 0.71428571 0.72857143 0.74285714 0.75714286 0.77142857 0.78571429 0.8 0.81428571 0.82857143 0.84285714 0.85714286 0.87142857 0.88571429 0.9 0.91428571 0.92857143 0.94285714 0.95714286 0.97142857 0.98571429 1 1 1 1 1 1
  arc A57 (9.2013, -31.6913) -> (11.1836, -31.0472) centre (0, 0) ccw
  spline S29 degree 5 poles (11.1751, -25.8812) (11.1807, -25.8942) (11.1916, -25.9204) (11.2069, -25.9601) (11.2252, -26.0137) (11.2454, -26.0818) (11.2636, -26.1506) (11.2806, -26.2198) (11.2969, -26.2893) (11.3128, -26.359) (11.3281, -26.4288) (11.3429, -26.4989) (11.3568, -26.5692) (11.3697, -26.6399) (11.3817, -26.7109) (11.3928, -26.7822) (11.4031, -26.8537) (11.4127, -26.9254) (11.4218, -26.9973) (11.4303, -27.0694) (11.4383, -27.1416) (11.4457, -27.214) (11.4525, -27.2866) (11.4587, -27.3593) (11.4643, -27.4322) (11.4693, -27.5053) (11.4737, -27.5785) (11.4776, -27.6519) (11.481, -27.7254) (11.4839, -27.799) (11.4863, -27.8727) (11.4881, -27.9466) (11.4895, -28.0206) (11.4904, -28.0947) (11.4908, -28.1689) (11.4907, -28.2433) (11.4901, -28.3177) (11.489, -28.3922) (11.4875, -28.4669) (11.4855, -28.5416) (11.4831, -28.6165) (11.4802, -28.6914) (11.4769, -28.7664) (11.4731, -28.8415) (11.4689, -28.9167) (11.4642, -28.992) (11.4591, -29.0673) (11.4536, -29.1427) (11.4477, -29.2182) (11.4413, -29.2938) (11.4345, -29.3695) (11.4273, -29.4452) (11.4196, -29.5209) (11.4116, -29.5968) (11.4032, -29.6727) (11.3943, -29.7486) (11.385, -29.8246) (11.3754, -29.9007) (11.3653, -29.9768) (11.3549, -30.053) (11.344, -30.1292) (11.3328, -30.2055) (11.3211, -30.2818) (11.3091, -30.3582) (11.2967, -30.4346) (11.2839, -30.511) (11.2707, -30.5875) (11.2572, -30.664) (11.2432, -30.7406) (11.2289, -30.8172) (11.2142, -30.8938) (11.2022, -30.9551) (11.193, -31.0011) (11.1867, -31.0318) (11.1836, -31.0472) knots 0 0 0 0 0 0 0.01428571 0.02857143 0.04285714 0.05714286 0.07142857 0.08571429 0.1 0.11428571 0.12857143 0.14285714 0.15714286 0.17142857 0.18571429 0.2 0.21428571 0.22857143 0.24285714 0.25714286 0.27142857 0.28571429 0.3 0.31428571 0.32857143 0.34285714 0.35714286 0.37142857 0.38571429 0.4 0.41428571 0.42857143 0.44285714 0.45714286 0.47142857 0.48571429 0.5 0.51428571 0.52857143 0.54285714 0.55714286 0.57142857 0.58571429 0.6 0.61428571 0.62857143 0.64285714 0.65714286 0.67142857 0.68571429 0.7 0.71428571 0.72857143 0.74285714 0.75714286 0.77142857 0.78571429 0.8 0.81428571 0.82857143 0.84285714 0.85714286 0.87142857 0.88571429 0.9 0.91428571 0.92857143 0.94285714 0.95714286 0.97142857 0.98571429 1 1 1 1 1 1
  line L29 (11.1751, -25.8812) -> (11.0563, -25.6057)
  arc A58 (11.803, -23.5578) -> (11.0563, -25.6057) centre (12.5141, -24.9771) ccw
  arc A59 (11.803, -23.5578) -> (12.1211, -23.3957) centre (0, 0) ccw
  arc A60 (14.2167, -23.9954) -> (12.1211, -23.3957) centre (12.8513, -24.8053) ccw
  line L30 (14.2167, -23.9954) -> (14.3698, -24.2534)
  spline S30 degree 5 poles (14.3698, -24.2534) (14.377, -24.2657) (14.3918, -24.2899) (14.4149, -24.3255) (14.4475, -24.3719) (14.4907, -24.4282) (14.5357, -24.4834) (14.5817, -24.5378) (14.6283, -24.5918) (14.6754, -24.6456) (14.7228, -24.6991) (14.7709, -24.7522) (14.8196, -24.8048) (14.8691, -24.8568) (14.9195, -24.9083) (14.9707, -24.9591) (15.0225, -25.0095) (15.0749, -25.0594) (15.1278, -25.109) (15.1811, -25.1583) (15.2348, -25.2072) (15.289, -25.2557) (15.3437, -25.3039) (15.3989, -25.3517) (15.4546, -25.399) (15.5108, -25.446) (15.5674, -25.4927) (15.6245, -25.5389) (15.6819, -25.5849) (15.7398, -25.6305) (15.7981, -25.6758) (15.8567, -25.7207) (15.9158, -25.7653) (15.9752, -25.8096) (16.035, -25.8535) (16.0952, -25.8971) (16.1558, -25.9404) (16.2167, -25.9834) (16.278, -26.026) (16.3396, -26.0683) (16.4016, -26.1104) (16.4639, -26.1521) (16.5266, -26.1935) (16.5896, -26.2346) (16.6529, -26.2753) (16.7165, -26.3158) (16.7804, -26.356) (16.8447, -26.3958) (16.9093, -26.4354) (16.9742, -26.4747) (17.0394, -26.5136) (17.1048, -26.5523) (17.1706, -26.5907) (17.2367, -26.6287) (17.3031, -26.6665) (17.3697, -26.704) (17.4367, -26.7412) (17.5039, -26.7781) (17.5714, -26.8147) (17.6392, -26.851) (17.7072, -26.887) (17.7755, -26.9227) (17.8441, -26.9582) (17.913, -26.9933) (17.9821, -27.0282) (18.0514, -27.0628) (18.1211, -27.0971) (18.1909, -27.1311) (18.2611, -27.1648) (18.3314, -27.1983) (18.4021, -27.2314) (18.4588, -27.2577) (18.5014, -27.2773) (18.5299, -27.2903) (18.5441, -27.2968) knots 0 0 0 0 0 0 0.01428571 0.02857143 0.04285714 0.05714286 0.07142857 0.08571429 0.1 0.11428571 0.12857143 0.14285714 0.15714286 0.17142857 0.18571429 0.2 0.21428571 0.22857143 0.24285714 0.25714286 0.27142857 0.28571429 0.3 0.31428571 0.32857143 0.34285714 0.35714286 0.37142857 0.38571429 0.4 0.41428571 0.42857143 0.44285714 0.45714286 0.47142857 0.48571429 0.5 0.51428571 0.52857143 0.54285714 0.55714286 0.57142857 0.58571429 0.6 0.61428571 0.62857143 0.64285714 0.65714286 0.67142857 0.68571429 0.7 0.71428571 0.72857143 0.74285714 0.75714286 0.77142857 0.78571429 0.8 0.81428571 0.82857143 0.84285714 0.85714286 0.87142857 0.88571429 0.9 0.91428571 0.92857143 0.94285714 0.95714286 0.97142857 0.98571429 1 1 1 1 1 1
  arc A61 (18.5441, -27.2968) -> (20.2304, -26.0717) centre (0, 0) ccw
  spline S31 degree 5 poles (18.6259, -21.1612) (18.6353, -21.1718) (18.6537, -21.1934) (18.6805, -21.2264) (18.7145, -21.2717) (18.7547, -21.3302) (18.7933, -21.39) (18.8308, -21.4506) (18.8678, -21.5117) (18.9044, -21.573) (18.9407, -21.6347) (18.9763, -21.6968) (19.0113, -21.7594) (19.0454, -21.8226) (19.0788, -21.8864) (19.1113, -21.9508) (19.1432, -22.0156) (19.1745, -22.0809) (19.2054, -22.1465) (19.2358, -22.2124) (19.2657, -22.2786) (19.2951, -22.3452) (19.324, -22.4121) (19.3523, -22.4793) (19.3802, -22.5469) (19.4075, -22.6149) (19.4344, -22.6832) (19.4607, -22.7517) (19.4867, -22.8206) (19.5122, -22.8897) (19.5372, -22.9591) (19.5618, -23.0288) (19.586, -23.0987) (19.6098, -23.1689) (19.6331, -23.2394) (19.6559, -23.3101) (19.6784, -23.3811) (19.7004, -23.4523) (19.722, -23.5238) (19.7432, -23.5955) (19.7641, -23.6674) (19.7845, -23.7396) (19.8045, -23.8119) (19.8241, -23.8845) (19.8433, -23.9573) (19.8621, -24.0304) (19.8806, -24.1036) (19.8986, -24.177) (19.9163, -24.2507) (19.9336, -24.3245) (19.9505, -24.3986) (19.967, -24.4728) (19.9832, -24.5472) (19.999, -24.6218) (20.0144, -24.6966) (20.0295, -24.7716) (20.0441, -24.8467) (20.0585, -24.9221) (20.0724, -24.9976) (20.086, -25.0733) (20.0992, -25.1491) (20.1121, -25.2251) (20.1246, -25.3013) (20.1368, -25.3776) (20.1486, -25.4541) (20.16, -25.5308) (20.1711, -25.6076) (20.1819, -25.6846) (20.1923, -25.7617) (20.2024, -25.839) (20.2121, -25.9164) (20.2196, -25.9784) (20.225, -26.025) (20.2286, -26.0561) (20.2304, -26.0717) knots 0 0 0 0 0 0 0.01428571 0.02857143 0.04285714 0.05714286 0.07142857 0.08571429 0.1 0.11428571 0.12857143 0.14285714 0.15714286 0.17142857 0.18571429 0.2 0.21428571 0.22857143 0.24285714 0.25714286 0.27142857 0.28571429 0.3 0.31428571 0.32857143 0.34285714 0.35714286 0.37142857 0.38571429 0.4 0.41428571 0.42857143 0.44285714 0.45714286 0.47142857 0.48571429 0.5 0.51428571 0.52857143 0.54285714 0.55714286 0.57142857 0.58571429 0.6 0.61428571 0.62857143 0.64285714 0.65714286 0.67142857 0.68571429 0.7 0.71428571 0.72857143 0.74285714 0.75714286 0.77142857 0.78571429 0.8 0.81428571 0.82857143 0.84285714 0.85714286 0.87142857 0.88571429 0.9 0.91428571 0.92857143 0.94285714 0.95714286 0.97142857 0.98571429 1 1 1 1 1 1
  line L31 (18.6259, -21.1612) -> (18.4278, -20.9359)
  arc A62 (18.5051, -18.7575) -> (18.4278, -20.9359) centre (19.62, -19.8876) ccw
  arc A63 (18.5051, -18.7575) -> (18.7575, -18.5051) centre (0, 0) ccw
  arc A64 (20.9359, -18.4278) -> (18.7575, -18.5051) centre (19.8876, -19.62) ccw
  line L32 (20.9359, -18.4278) -> (21.1612, -18.6259)
  spline S32 degree 5 poles (21.1612, -18.6259) (21.1718, -18.6353) (21.1934, -18.6537) (21.2264, -18.6805) (21.2717, -18.7145) (21.3302, -18.7547) (21.39, -18.7933) (21.4506, -18.8308) (21.5117, -18.8678) (21.573, -18.9044) (21.6347, -18.9407) (21.6968, -18.9763) (21.7594, -19.0113) (21.8226, -19.0454) (21.8864, -19.0788) (21.9508, -19.1113) (22.0156, -19.1432) (22.0809, -19.1745) (22.1465, -19.2054) (22.2124, -19.2358) (22.2786, -19.2657) (22.3452, -19.2951) (22.4121, -19.324) (22.4793, -19.3523) (22.5469, -19.3802) (22.6149, -19.4075) (22.6832, -19.4344) (22.7517, -19.4607) (22.8206, -19.4867) (22.8897, -19.5122) (22.9591, -19.5372) (23.0288, -19.5618) (23.0987, -19.586) (23.1689, -19.6098) (23.2394, -19.6331) (23.3101, -19.6559) (23.3811, -19.6784) (23.4523, -19.7004) (23.5238, -19.722) (23.5955, -19.7432) (23.6674, -19.7641) (23.7396, -19.7845) (23.8119, -19.8045) (23.8845, -19.8241) (23.9573, -19.8433) (24.0304, -19.8621) (24.1036, -19.8806) (24.177, -19.8986) (24.2507, -19.9163) (24.3245, -19.9336) (24.3986, -19.9505) (24.4728, -19.967) (24.5472, -19.9832) (24.6218, -19.999) (24.6966, -20.0144) (24.7716, -20.0295) (24.8467, -20.0441) (24.9221, -20.0585) (24.9976, -20.0724) (25.0733, -20.086) (25.1491, -20.0992) (25.2251, -20.1121) (25.3013, -20.1246) (25.3776, -20.1368) (25.4541, -20.1486) (25.5308, -20.16) (25.6076, -20.1711) (25.6846, -20.1819) (25.7617, -20.1923) (25.839, -20.2024) (25.9164, -20.2121) (25.9784, -20.2196) (26.025, -20.225) (26.0561, -20.2286) (26.0717, -20.2304) knots 0 0 0 0 0 0 0.01428571 0.02857143 0.04285714 0.05714286 0.07142857 0.08571429 0.1 0.11428571 0.12857143 0.14285714 0.15714286 0.17142857 0.18571429 0.2 0.21428571 0.22857143 0.24285714 0.25714286 0.27142857 0.28571429 0.3 0.31428571 0.32857143 0.34285714 0.35714286 0.37142857 0.38571429 0.4 0.41428571 0.42857143 0.44285714 0.45714286 0.47142857 0.48571429 0.5 0.51428571 0.52857143 0.54285714 0.55714286 0.57142857 0.58571429 0.6 0.61428571 0.62857143 0.64285714 0.65714286 0.67142857 0.68571429 0.7 0.71428571 0.72857143 0.74285714 0.75714286 0.77142857 0.78571429 0.8 0.81428571 0.82857143 0.84285714 0.85714286 0.87142857 0.88571429 0.9 0.91428571 0.92857143 0.94285714 0.95714286 0.97142857 0.98571429 1 1 1 1 1 1
  arc A65 (26.0717, -20.2304) -> (27.2968, -18.5441) centre (0, 0) ccw
  spline S33 degree 5 poles (24.2534, -14.3698) (24.2657, -14.377) (24.2899, -14.3918) (24.3255, -14.4149) (24.3719, -14.4475) (24.4282, -14.4907) (24.4834, -14.5357) (24.5378, -14.5817) (24.5918, -14.6283) (24.6456, -14.6754) (24.6991, -14.7228) (24.7522, -14.7709) (24.8048, -14.8196) (24.8568, -14.8691) (24.9083, -14.9195) (24.9591, -14.9707) (25.0095, -15.0225) (25.0594, -15.0749) (25.109, -15.1278) (25.1583, -15.1811) (25.2072, -15.2348) (25.2557, -15.289) (25.3039, -15.3437) (25.3517, -15.3989) (25.399, -15.4546) (25.446, -15.5108) (25.4927, -15.5674) (25.5389, -15.6245) (25.5849, -15.6819) (25.6305, -15.7398) (25.6758, -15.7981) (25.7207, -15.8567) (25.7653, -15.9158) (25.8096, -15.9752) (25.8535, -16.035) (25.8971, -16.0952) (25.9404, -16.1558) (25.9834, -16.2167) (26.026, -16.278) (26.0683, -16.3396) (26.1104, -16.4016) (26.1521, -16.4639) (26.1935, -16.5266) (26.2346, -16.5896) (26.2753, -16.6529) (26.3158, -16.7165) (26.356, -16.7804) (26.3958, -16.8447) (26.4354, -16.9093) (26.4747, -16.9742) (26.5136, -17.0394) (26.5523, -17.1048) (26.5907, -17.1706) (26.6287, -17.2367) (26.6665, -17.3031) (26.704, -17.3697) (26.7412, -17.4367) (26.7781, -17.5039) (26.8147, -17.5714) (26.851, -17.6392) (26.887, -17.7072) (26.9227, -17.7755) (26.9582, -17.8441) (26.9933, -17.913) (27.0282, -17.9821) (27.0628, -18.0514) (27.0971, -18.1211) (27.1311, -18.1909) (27.1648, -18.2611) (27.1983, -18.3314) (27.2314, -18.4021) (27.2577, -18.4588) (27.2773, -18.5014) (27.2903, -18.5299) (27.2968, -18.5441) knots 0 0 0 0 0 0 0.01428571 0.02857143 0.04285714 0.05714286 0.07142857 0.08571429 0.1 0.11428571 0.12857143 0.14285714 0.15714286 0.17142857 0.18571429 0.2 0.21428571 0.22857143 0.24285714 0.25714286 0.27142857 0.28571429 0.3 0.31428571 0.32857143 0.34285714 0.35714286 0.37142857 0.38571429 0.4 0.41428571 0.42857143 0.44285714 0.45714286 0.47142857 0.48571429 0.5 0.51428571 0.52857143 0.54285714 0.55714286 0.57142857 0.58571429 0.6 0.61428571 0.62857143 0.64285714 0.65714286 0.67142857 0.68571429 0.7 0.71428571 0.72857143 0.74285714 0.75714286 0.77142857 0.78571429 0.8 0.81428571 0.82857143 0.84285714 0.85714286 0.87142857 0.88571429 0.9 0.91428571 0.92857143 0.94285714 0.95714286 0.97142857 0.98571429 1 1 1 1 1 1
  line L33 (24.2534, -14.3698) -> (23.9954, -14.2167)
  arc A66 (23.3957, -12.1211) -> (23.9954, -14.2167) centre (24.8053, -12.8513) ccw
  arc A67 (23.3957, -12.1211) -> (23.5578, -11.803) centre (0, 0) ccw
  arc A68 (25.6057, -11.0563) -> (23.5578, -11.803) centre (24.9771, -12.5141) ccw
  line L34 (25.6057, -11.0563) -> (25.8812, -11.1751)
  spline S34 degree 5 poles (25.8812, -11.1751) (25.8942, -11.1807) (25.9204, -11.1916) (25.9601, -11.2069) (26.0137, -11.2252) (26.0818, -11.2454) (26.1506, -11.2636) (26.2198, -11.2806) (26.2893, -11.2969) (26.359, -11.3128) (26.4288, -11.3281) (26.4989, -11.3429) (26.5692, -11.3568) (26.6399, -11.3697) (26.7109, -11.3817) (26.7822, -11.3928) (26.8537, -11.4031) (26.9254, -11.4127) (26.9973, -11.4218) (27.0694, -11.4303) (27.1416, -11.4383) (27.214, -11.4457) (27.2866, -11.4525) (27.3593, -11.4587) (27.4322, -11.4643) (27.5053, -11.4693) (27.5785, -11.4737) (27.6519, -11.4776) (27.7254, -11.481) (27.799, -11.4839) (27.8727, -11.4863) (27.9466, -11.4881) (28.0206, -11.4895) (28.0947, -11.4904) (28.1689, -11.4908) (28.2433, -11.4907) (28.3177, -11.4901) (28.3922, -11.489) (28.4669, -11.4875) (28.5416, -11.4855) (28.6165, -11.4831) (28.6914, -11.4802) (28.7664, -11.4769) (28.8415, -11.4731) (28.9167, -11.4689) (28.992, -11.4642) (29.0673, -11.4591) (29.1427, -11.4536) (29.2182, -11.4477) (29.2938, -11.4413) (29.3695, -11.4345) (29.4452, -11.4273) (29.5209, -11.4196) (29.5968, -11.4116) (29.6727, -11.4032) (29.7486, -11.3943) (29.8246, -11.385) (29.9007, -11.3754) (29.9768, -11.3653) (30.053, -11.3549) (30.1292, -11.344) (30.2055, -11.3328) (30.2818, -11.3211) (30.3582, -11.3091) (30.4346, -11.2967) (30.511, -11.2839) (30.5875, -11.2707) (30.664, -11.2572) (30.7406, -11.2432) (30.8172, -11.2289) (30.8938, -11.2142) (30.9551, -11.2022) (31.0011, -11.193) (31.0318, -11.1867) (31.0472, -11.1836) knots 0 0 0 0 0 0 0.01428571 0.02857143 0.04285714 0.05714286 0.07142857 0.08571429 0.1 0.11428571 0.12857143 0.14285714 0.15714286 0.17142857 0.18571429 0.2 0.21428571 0.22857143 0.24285714 0.25714286 0.27142857 0.28571429 0.3 0.31428571 0.32857143 0.34285714 0.35714286 0.37142857 0.38571429 0.4 0.41428571 0.42857143 0.44285714 0.45714286 0.47142857 0.48571429 0.5 0.51428571 0.52857143 0.54285714 0.55714286 0.57142857 0.58571429 0.6 0.61428571 0.62857143 0.64285714 0.65714286 0.67142857 0.68571429 0.7 0.71428571 0.72857143 0.74285714 0.75714286 0.77142857 0.78571429 0.8 0.81428571 0.82857143 0.84285714 0.85714286 0.87142857 0.88571429 0.9 0.91428571 0.92857143 0.94285714 0.95714286 0.97142857 0.98571429 1 1 1 1 1 1
  arc A69 (31.0472, -11.1836) -> (31.6913, -9.2013) centre (0, 0) ccw
  spline S35 degree 5 poles (27.5069, -6.1717) (27.5207, -6.1748) (27.5483, -6.1814) (27.5894, -6.1924) (27.6436, -6.2091) (27.7105, -6.2328) (27.7768, -6.2585) (27.8428, -6.2854) (27.9086, -6.3131) (27.9743, -6.3412) (28.0399, -6.3698) (28.1052, -6.3991) (28.1703, -6.4291) (28.2351, -6.4602) (28.2996, -6.4923) (28.3637, -6.5252) (28.4276, -6.5589) (28.4913, -6.5933) (28.5548, -6.6282) (28.6182, -6.6637) (28.6813, -6.6997) (28.7442, -6.7362) (28.8069, -6.7734) (28.8694, -6.8111) (28.9317, -6.8495) (28.9937, -6.8884) (29.0556, -6.9278) (29.1172, -6.9678) (29.1786, -7.0083) (29.2399, -7.0492) (29.301, -7.0906) (29.3618, -7.1325) (29.4225, -7.1749) (29.483, -7.2177) (29.5432, -7.261) (29.6033, -7.3048) (29.6632, -7.3491) (29.7229, -7.3937) (29.7824, -7.4388) (29.8417, -7.4844) (29.9008, -7.5303) (29.9597, -7.5767) (30.0185, -7.6235) (30.077, -7.6707) (30.1353, -7.7183) (30.1935, -7.7663) (30.2515, -7.8147) (30.3092, -7.8635) (30.3668, -7.9127) (30.4242, -7.9623) (30.4814, -8.0122) (30.5384, -8.0626) (30.5952, -8.1133) (30.6519, -8.1644) (30.7083, -8.2158) (30.7645, -8.2676) (30.8206, -8.3198) (30.8765, -8.3723) (30.9321, -8.4252) (30.9876, -8.4784) (31.0429, -8.532) (31.098, -8.5859) (31.1529, -8.6402) (31.2076, -8.6948) (31.2621, -8.7498) (31.3164, -8.8051) (31.3706, -8.8607) (31.4245, -8.9166) (31.4783, -8.9729) (31.5318, -9.0295) (31.5852, -9.0864) (31.6277, -9.1322) (31.6595, -9.1667) (31.6807, -9.1898) (31.6913, -9.2013) knots 0 0 0 0 0 0 0.01428571 0.02857143 0.04285714 0.05714286 0.07142857 0.08571429 0.1 0.11428571 0.12857143 0.14285714 0.15714286 0.17142857 0.18571429 0.2 0.21428571 0.22857143 0.24285714 0.25714286 0.27142857 0.28571429 0.3 0.31428571 0.32857143 0.34285714 0.35714286 0.37142857 0.38571429 0.4 0.41428571 0.42857143 0.44285714 0.45714286 0.47142857 0.48571429 0.5 0.51428571 0.52857143 0.54285714 0.55714286 0.57142857 0.58571429 0.6 0.61428571 0.62857143 0.64285714 0.65714286 0.67142857 0.68571429 0.7 0.71428571 0.72857143 0.74285714 0.75714286 0.77142857 0.78571429 0.8 0.81428571 0.82857143 0.84285714 0.85714286 0.87142857 0.88571429 0.9 0.91428571 0.92857143 0.94285714 0.95714286 0.97142857 0.98571429 1 1 1 1 1 1
  line L35 (27.5069, -6.1717) -> (27.2142, -6.1059)
  arc A70 (25.9963, -4.2981) -> (27.2142, -6.1059) centre (27.5625, -4.5571) ccw
  arc A71 (25.9963, -4.2981) -> (26.0521, -3.9455) centre (0, 0) ccw
  arc A72 (27.7691, -2.6026) -> (26.0521, -3.9455) centre (27.6217, -4.1832) ccw
  line L36 (27.7691, -2.6026) -> (28.0678, -2.6304)
  spline S36 degree 5 poles (28.0678, -2.6304) (28.0819, -2.6317) (28.1102, -2.634) (28.1526, -2.6363) (28.2093, -2.6371) (28.2803, -2.6353) (28.3513, -2.6314) (28.4224, -2.6261) (28.4935, -2.6201) (28.5647, -2.6137) (28.6359, -2.6067) (28.7071, -2.5991) (28.7783, -2.5906) (28.8495, -2.5811) (28.9207, -2.5705) (28.9919, -2.559) (29.0631, -2.5467) (29.1343, -2.5337) (29.2055, -2.5201) (29.2767, -2.5059) (29.3478, -2.4912) (29.419, -2.4759) (29.4901, -2.46) (29.5612, -2.4434) (29.6322, -2.4261) (29.7033, -2.4083) (29.7743, -2.3899) (29.8453, -2.3709) (29.9162, -2.3515) (29.9871, -2.3314) (30.058, -2.3109) (30.1288, -2.2899) (30.1996, -2.2683) (30.2704, -2.2463) (30.3411, -2.2237) (30.4117, -2.2006) (30.4824, -2.1771) (30.5529, -2.153) (30.6235, -2.1285) (30.6939, -2.1035) (30.7644, -2.0781) (30.8347, -2.0522) (30.905, -2.0259) (30.9753, -1.9991) (31.0455, -1.9718) (31.1156, -1.9441) (31.1857, -1.916) (31.2558, -1.8874) (31.3257, -1.8584) (31.3956, -1.829) (31.4655, -1.7992) (31.5352, -1.7689) (31.6049, -1.7383) (31.6746, -1.7072) (31.7442, -1.6757) (31.8137, -1.6438) (31.8831, -1.6115) (31.9524, -1.5788) (32.0217, -1.5457) (32.0909, -1.5122) (32.1601, -1.4784) (32.2291, -1.4441) (32.2981, -1.4094) (32.367, -1.3744) (32.4359, -1.339) (32.5046, -1.3032) (32.5733, -1.267) (32.6419, -1.2305) (32.7104, -1.1936) (32.7788, -1.1563) (32.8471, -1.1186) (32.9017, -1.0882) (32.9427, -1.0652) (32.9699, -1.0499) (32.9835, -1.0421) knots 0 0 0 0 0 0 0.01428571 0.02857143 0.04285714 0.05714286 0.07142857 0.08571429 0.1 0.11428571 0.12857143 0.14285714 0.15714286 0.17142857 0.18571429 0.2 0.21428571 0.22857143 0.24285714 0.25714286 0.27142857 0.28571429 0.3 0.31428571 0.32857143 0.34285714 0.35714286 0.37142857 0.38571429 0.4 0.41428571 0.42857143 0.44285714 0.45714286 0.47142857 0.48571429 0.5 0.51428571 0.52857143 0.54285714 0.55714286 0.57142857 0.58571429 0.6 0.61428571 0.62857143 0.64285714 0.65714286 0.67142857 0.68571429 0.7 0.71428571 0.72857143 0.74285714 0.75714286 0.77142857 0.78571429 0.8 0.81428571 0.82857143 0.84285714 0.85714286 0.87142857 0.88571429 0.9 0.91428571 0.92857143 0.94285714 0.95714286 0.97142857 0.98571429 1 1 1 1 1 1
  arc A73 (32.9835, -1.0421) -> (32.9835, 1.0421) centre (0, 0) ccw